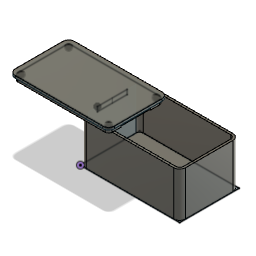
DoorSwitch (Autodesk Fusion 360 design; units mm, degrees)
Autodesk Fusion 360 part; units mm, degrees
sketch "Base" plane through (0, 0, 0) normal (0, 1, 0) x (1, 0, 0) in component "Top"
  line L0 (0, 0) -> (67, 0)
  line L1 (67, 0) -> (67, 40)
  line L2 (67, 40) -> (0, 40)
  line L3 (0, 40) -> (0, 0)
  dimension "d6" = 67
  dimension "d7" = 40
  constraint horizontal L0
  constraint vertical L1
  constraint horizontal L2
  constraint vertical L3
  constraint coincident L0.start L3.end
  measures "d6" distance of L0.start L0.end
  measures "d7" distance of L0.start L2.end
extrude "Extrude1" add sketch "Base" along normal blind 30 makes body 1 in component "Top"
fillet "Fillet1" radius 4 4 edges at (67, 15, 0) (0, 15, 0) (67, 15, -40) (0, 15, -40) on bodies 1 in component "Top"
shell "Shell1" thickness 1.5 removed faces 1 at (43.3333, 30, -13.3333) on bodies 1 in component "Top"
sketch "Knob" plane through (1.5, 0, 0) normal (1, 0, 0) x (0, 0, -1) in component "Top"
  line L0 (36, 1.5) -> (36, 30)
  line L1 (36, 30) -> (4, 30)
  line L2 (4, 30) -> (4, 1.5)
  line L3 (4, 1.5) -> (36, 1.5)
  line L4 (10, 30) -> (30, 30)
  line L5 (30, 30) -> (30, 27)
  line L6 (30, 27) -> (10, 27)
  line L7 (10, 27) -> (10, 30)
  line L8 (20, 30) -> (20, 27) construction
  dimension "d12" = 20
  dimension "d13" = 3
  constraint horizontal L4
  constraint vertical L5
  constraint horizontal L6
  constraint vertical L7
  constraint coincident L1 L4.start
  constraint midpoint L1 L8.start
  constraint midpoint L6 L8.end
  constraint vertical L8
  measures "d12" distance of L5.end L6.end
  measures "d13" distance of L4.end L5.end
extrude "Extrude2" add sketch "Knob" along normal blind 6 draft -45 contours L1 L4 L5 L6 L7 bodies 1 in component "Top"
ref_plane "WorkPlane2" through (33.5, 15, -20) normal (-1, 0, 0) x (0, 0, 1) in component "Top"
mirror "Mirror1" about plane through (33.5, 15, -20) normal (-1, 0, 0) of "Extrude2" in component "Top"
sketch "Top" plane through (0, 30, 0) normal (0, 1, 0) x (-1, 0, 0) in component "Base"
  line L0 (-67, -4) -> (-67, -36)
  arc A0 (-67, -36) -> (-63, -40) centre (-63, -36) ccw
  line L1 (-63, -40) -> (-4, -40)
  arc A1 (-4, -40) -> (0, -36) centre (-4, -36) ccw
  line L2 (0, -36) -> (0, -4)
  arc A2 (0, -4) -> (-4, 0) centre (-4, -4) ccw
  line L3 (-4, 0) -> (-63, 0)
  arc A3 (-63, 0) -> (-67, -4) centre (-63, -4) ccw
  line L4 (-65.5, -10) -> (-65.5, -4)
  arc A4 (-63, -1.5) -> (-65.5, -4) centre (-63, -4) ccw
  line L5 (-63, -1.5) -> (-4, -1.5)
  arc A5 (-1.5, -4) -> (-4, -1.5) centre (-4, -4) ccw
  line L6 (-1.5, -4) -> (-1.5, -10)
  line L7 (-1.5, -10) -> (-1.5, -30)
  line L8 (-1.5, -30) -> (-1.5, -36)
  arc A6 (-4, -38.5) -> (-1.5, -36) centre (-4, -36) ccw
  line L9 (-4, -38.5) -> (-63, -38.5)
  arc A7 (-65.5, -36) -> (-63, -38.5) centre (-63, -36) ccw
  line L10 (-65.5, -36) -> (-65.5, -30)
  line L11 (-65.5, -30) -> (-65.5, -10)
extrude "Extrude1'" add sketch "Top" along normal blind 1.5 separate body contours L0 A0 L1 A1 L2 A2 L3 A3 | L4 A4 L5 A5 L6 L7 L8 A6 L9 A7 L10 L11 makes body 2 in component "Base"
sketch "Lip" plane through (0, 30, 0) normal (0, -1, 0) x (1, 0, 0) in component "Base"
  arc A0 (67, -4) -> (63, 0) centre (63, -4) ccw
  line L0 (63, 0) -> (4, 0)
  arc A1 (4, 0) -> (0, -4) centre (4, -4) ccw
  line L1 (0, -4) -> (0, -36)
  arc A2 (0, -36) -> (4, -40) centre (4, -36) ccw
  line L2 (4, -40) -> (63, -40)
  arc A3 (63, -40) -> (67, -36) centre (63, -36) ccw
  line L3 (67, -36) -> (67, -4)
  line L4 (65.3, -36) -> (65.3, -4)
  arc A4 (65.3, -4) -> (63, -1.7) centre (63, -4) ccw
  line L5 (63, -1.7) -> (4, -1.7)
  arc A5 (4, -1.7) -> (1.7, -4) centre (4, -4) ccw
  line L6 (1.7, -4) -> (1.7, -36)
  arc A6 (1.7, -36) -> (4, -38.3) centre (4, -36) ccw
  line L7 (4, -38.3) -> (63, -38.3)
  arc A7 (63, -38.3) -> (65.3, -36) centre (63, -36) ccw
  dimension "d19" = 1.7
extrude "Extrude2'" add sketch "Lip" along normal blind 3 contours L4 A4 L5 A5 L6 A6 L7 A7 bodies 2 in component "Base"
extrude "Extrude3" cut sketch "Knob" along normal blind 3 draft -45 from surface at 0.2 contours L1 L4 L5 L6 L7 bodies 2 in component "Base"
mirror "Mirror1'" about plane through (33.5, 15, -20) normal (-1, 0, 0) of "Extrude3" in component "Base"
shell "Shell1'" thickness 1.5 removed faces 1 at (22.9, 27, -23.3333) on bodies 2 in component "Base"
chamfer "Chamfer1" distance 0.6 angle 45 2 edges at (1.7, 27, -20) (65.3, 27, -20) on bodies 2 in component "Base"
component "Enclosure" placed x (1, 0, 0) y (0, 1, 0) z (0, 0, 1) at (0, 0, 0)
component "Top" placed x (1, 0, 0) y (0, 1, 0) z (0, 0, 1) at (0, 0, 0) in component "Enclosure"
component "Base" placed x (1, 0, 0) y (0, 1, 0) z (0, 0, 1) at (0, 0, 0) in component "Enclosure"
equation "Width = 40 mm"
equation "length = 67 mm"
equation "heigth = 30 mm"
equation "shell = 1.5 mm"
equation "gap = 0.2 mm"
equation "d6 = length"
equation "d7 = Width"
equation "d8 = heigth"
equation "d11 = shell"
equation "d12 = Width / 2"
equation "d13 = shell * 2"
equation "d17 = shell"
equation "d19 = shell + gap"
equation "d20 = shell * 2"
equation "d23 = shell * 2"
equation "d26 = shell"
